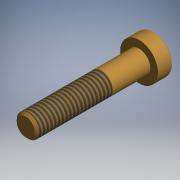
# Autodesk Inventor part: Zyl.Schr-M6x30_Stahl_X094085
Saved by Autodesk Inventor 2021 (Build 250183000, 183)
## iProperties
Part Number: Zyl.Schr-M6x30_Stahl_X094085
Material: Generic
Catalog Web Link: www.cadenas.de
Description: ZylSchraube DIN EN ISO 7984-Normalien
Vendor: ROSEKRIEGER
Document SubType Name: Modeling
Designer: partserver
Manufacturer: ROSEKRIEGER
Mass: 1.10201 g
Surface Area: 8.89539 cm^2
Volume: 1.10201 cm^3
Density: 1 g/cm^3
Appearance: PSOLRGB-203-152-72
Category: PARTsolutions
Company: ROSEKRIEGER
PSOL_IDENT_0: {$CADENAS_DATA\23d-libs\rose_krieger\pool_normalien\schrauben_scheiben_muttern\zyl_isk_din7984.prj},
PSOL_IDENT_1: 218 {VTYP=3D},{NB=Zyl.Schr-M6x30_Stahl_X094085},{LINA=Zyl.Schr-M6x30_Stahl_X094085},{NN=ZylSchraube
PSOL_IDENT_2: DIN EN ISO 7984},{DATE=25.02.2021 18:00:30},{GEOMDATE=11.12.2020 13:50:00},{VERSION=},{LINEID=900},{
PSOL_IDENT_3: WBVAR=},{WBNUMERIC=}  {NB=Zyl.Schr-M6x30_Stahl_X094085},{LINA=Zyl.Schr-M6x30_Stahl_X094085},{KT=DUMM
PSOL_IDENT_4: Y},{IDNR=},{ARTIKEL=Zylinderschraube},{TYPE=M6},{FNENN=6.000},{L=30.000},{NORM=DIN7984},{NORMALT=DIN
PSOL_IDENT_5: 7984},{BEST=X094085},{RKMATNR=X094085},{WERKSTOFFBEZ=Stahl},{WERKSTOFF=0},{OBERFLAECHE=1},{FKKL=8.8}
PSOL_IDENT_6: ,{KHOE=4.000},{KD=10.000},{B=20.000},{SW=4.000},{R=0.500},{TSS=4.000},{WARENNUMMER=73181569}
NB: Zyl.Schr-M6x30_Stahl_X094085
NN: ZylSchraube DIN EN ISO 7984
NT: Normalien
NBSYN: Zyl.Schr-$TYPE.x$L._$WERKSTOFFBEZ._$RKMATNR.
LINA: Zyl.Schr-M6x30_Stahl_X094085
CATALOG: RK Rose+Krieger
ARTIKEL: Zylinderschraube
TYPE: M6
FNENN: 6
L: 30
NORM: DIN7984
NORMALT: DIN7984
BEST: X094085
RKMATNR: X094085
WERKSTOFFBEZ: Stahl
WERKSTOFF: 0
OBERFLAECHE: 1
FKKL: 8.8
KHOE: 4
KD: 10
B: 20
SW: 4
R: 0.5
TSS: 4
WARENNUMMER: 73181569
SUPPLIER: ROSEKRIEGER
ARTICLENO: Zyl.Schr-M6x30_Stahl_X094085
BOMINFO: Zyl.Schr-M6x30_Stahl_X094085
CREATOR: CADENAS GmbH
Title: Zyl.Schr-M6x30_Stahl_X094085
Author: Cadenas PARTsolutions
Comments: Normalien
Autodesk Inventor part; units mm, degrees
ref_plane "Deaktiviert_NICHT_mehrverwenden_Zyl__Schraube_DIN_EN_ISO_4762_XY" through (0, 0, 0) normal (0, 1, 0) x (1, 0, 0)
ref_plane "Deaktiviert_NICHT_mehrverwenden_Zyl__Schraube_DIN_EN_ISO_4762_YZ" through (0, 0, 0) normal (1, 0, 0) x (0, 0, -1)
ref_plane "Deaktiviert_NICHT_mehrverwenden_Zyl__Schraube_DIN_EN_ISO_4762_ZX" through (0, 0, 0) normal (0, 0, -1) x (0, 1, 0)
sketch "Skizze_1" plane through (0, 0, 0) normal (0, 0, 1) x (1, 0, 0)
  line L0 (0, -30) -> (0, 0)
  line L1 (0, 0) -> (3, 0)
  line L2 (3, 0) -> (3, -29.3865)
  line L3 (3, -29.3865) -> (2.3865, -30)
  line L4 (2.3865, -30) -> (0, -30)
  line L5 (0, -30) -> (0, 0)
  constraints: 12 end point
revolve "Revolution1" add sketch "Skizze_1" angle 360 about axis through (0, -30, 0) along (0, -1, 0)
thread "Thread1" size "M6x1" class "6g" standard "ISO Metric profile" length 19.3865
sketch "Skizze_2" plane through (0, 0, 0) normal (0, 0, 1) x (1, 0, 0)
  line L0 (0, 0) -> (0, 4)
  line L1 (0, 4) -> (4.5, 4)
  arc A0 (5, 3.5) -> (4.5, 4) centre (4.5, 3.5) ccw
  line L2 (5, 3.5) -> (5, 0)
  line L3 (5, 0) -> (0, 0)
  line L4 (0, 0) -> (0, 4)
  constraints: 10 end point, 2 point on circle, 1 centre point
revolve "Revolution2" add sketch "Skizze_2" angle 360 about axis through (0, 0, 0) along (0, -1, 0)
sketch "Skizze_3" plane through (0, 4, 0) normal (0, 1, 0) x (1, 0, 0)
  line L0 (-2, -1.1547) -> (0, -2.3094)
  line L1 (0, -2.3094) -> (2, -1.1547)
  line L2 (2, -1.1547) -> (2, 1.1547)
  line L3 (2, 1.1547) -> (0, 2.3094)
  line L4 (0, 2.3094) -> (-2, 1.1547)
  line L5 (-2, 1.1547) -> (-2, -1.1547)
  constraints: 12 end point
extrude "Extrusion1" cut sketch "Skizze_3" against normal blind 4
ref_plane "EP_XY" through (0, 0, 0) normal (0, 1, 0) x (1, 0, 0)
ref_plane "EP_YZ" through (0, 0, 0) normal (1, 0, 0) x (0, 0, -1)
ref_plane "EP_ZX" through (0, 0, 0) normal (0, 0, -1) x (0, 1, 0)
ref_plane "EP_Schraube_XY" through (0, 0, 0) normal (0, 1, 0) x (1, 0, 0)
ref_plane "EP_Schraube_YZ" through (0, 0, 0) normal (1, 0, 0) x (0, 0, -1)
ref_plane "EP_Schraube_ZX" through (0, 0, 0) normal (0, 0, -1) x (0, 1, 0)
body "Solid1"
